Autodesk Fusion 360 part; units mm, degrees
(part 7 of 7)
  spline S25 degree 3 poles (-97.5, 187.4565) (-97.1129, 187.1804) (-96.7258, 186.9044) (-96.3387, 186.6283) (-94.9048, 185.6057) (-93.8881, 184.0523) (-93.1468, 182.2521) (-92.4554, 180.5733) (-91.9675, 178.6373) (-91.4195, 176.7225) (-91.0808, 175.5389) (-90.7149, 174.3638) (-90.3326, 173.4325) (-90.2208, 173.1603) (-90.1088, 172.9111) (-90, 172.6931) knots -1.056001 -1.056001 -1.056001 -1.056001 -1 -1 -1 -0.851292 -0.851292 -0.851292 -0.71262 -0.71262 -0.71262 -0.626906 -0.626906 -0.626906 -0.601856 -0.601856 -0.601856 -0.601856
  spline S26 degree 3 poles (-90, 172.6931) (-89.5881, 173.5183) (-89.1514, 174.7828) (-88.7668, 176.0817) (-88.2129, 177.9522) (-87.737, 179.9069) (-87.1002, 181.6203) (-86.4085, 183.4814) (-85.486, 185.1149) (-84.1355, 186.2591) (-83.9823, 186.3889) (-83.8242, 186.5122) (-83.6613, 186.6283) (-83.2742, 186.9044) (-82.8871, 187.1804) (-82.5, 187.4565) knots -0.398144 -0.398144 -0.398144 -0.398144 -0.30293 -0.30293 -0.30293 -0.165823 -0.165823 -0.165823 -0.016893 -0.016893 -0.016893 0 0 0 0.056001 0.056001 0.056001 0.056001
  spline S27 degree 3 poles (-82.5, 187.4565) (-82.1129, 187.1804) (-81.7258, 186.9044) (-81.3387, 186.6283) (-79.9048, 185.6057) (-78.8881, 184.0523) (-78.1468, 182.2521) (-77.4554, 180.5733) (-76.9675, 178.6373) (-76.4195, 176.7225) (-76.0808, 175.5389) (-75.7149, 174.3638) (-75.3326, 173.4325) (-75.2208, 173.1603) (-75.1088, 172.9111) (-75, 172.6931) knots -1.056001 -1.056001 -1.056001 -1.056001 -1 -1 -1 -0.851292 -0.851292 -0.851292 -0.71262 -0.71262 -0.71262 -0.626906 -0.626906 -0.626906 -0.601856 -0.601856 -0.601856 -0.601856
  spline S28 degree 3 poles (-75, 172.6931) (-74.5881, 173.5183) (-74.1514, 174.7828) (-73.7668, 176.0817) (-73.2129, 177.9522) (-72.737, 179.9069) (-72.1002, 181.6203) (-71.4085, 183.4814) (-70.486, 185.1149) (-69.1355, 186.2591) (-68.9823, 186.3889) (-68.8242, 186.5122) (-68.6613, 186.6283) (-68.2742, 186.9044) (-67.8871, 187.1804) (-67.5, 187.4565) knots -0.398144 -0.398144 -0.398144 -0.398144 -0.30293 -0.30293 -0.30293 -0.165823 -0.165823 -0.165823 -0.016893 -0.016893 -0.016893 0 0 0 0.056001 0.056001 0.056001 0.056001
  spline S29 degree 3 poles (-67.5, 187.4565) (-67.1129, 187.1804) (-66.7258, 186.9044) (-66.3387, 186.6283) (-64.9048, 185.6057) (-63.8881, 184.0523) (-63.1468, 182.2521) (-62.4554, 180.5733) (-61.9675, 178.6373) (-61.4195, 176.7225) (-61.0808, 175.5389) (-60.7149, 174.3638) (-60.3326, 173.4325) (-60.2208, 173.1603) (-60.1088, 172.9111) (-60, 172.6931) knots -1.056001 -1.056001 -1.056001 -1.056001 -1 -1 -1 -0.851292 -0.851292 -0.851292 -0.71262 -0.71262 -0.71262 -0.626906 -0.626906 -0.626906 -0.601856 -0.601856 -0.601856 -0.601856
  spline S30 degree 3 poles (-60, 172.6931) (-59.5881, 173.5183) (-59.1514, 174.7828) (-58.7668, 176.0817) (-58.2129, 177.9522) (-57.737, 179.9069) (-57.1002, 181.6203) (-56.4085, 183.4814) (-55.486, 185.1149) (-54.1355, 186.2591) (-53.9823, 186.3889) (-53.8242, 186.5122) (-53.6613, 186.6283) (-53.2742, 186.9044) (-52.8871, 187.1804) (-52.5, 187.4565) knots -0.398144 -0.398144 -0.398144 -0.398144 -0.30293 -0.30293 -0.30293 -0.165823 -0.165823 -0.165823 -0.016893 -0.016893 -0.016893 0 0 0 0.056001 0.056001 0.056001 0.056001
  spline S31 degree 3 poles (-52.5, 187.4565) (-52.1129, 187.1804) (-51.7258, 186.9044) (-51.3387, 186.6283) (-49.9048, 185.6057) (-48.8881, 184.0523) (-48.1468, 182.2521) (-47.4554, 180.5733) (-46.9675, 178.6373) (-46.4195, 176.7225) (-46.0808, 175.5389) (-45.7149, 174.3638) (-45.3326, 173.4325) (-45.2208, 173.1603) (-45.1088, 172.9111) (-45, 172.6931) knots -1.056001 -1.056001 -1.056001 -1.056001 -1 -1 -1 -0.851292 -0.851292 -0.851292 -0.71262 -0.71262 -0.71262 -0.626906 -0.626906 -0.626906 -0.601856 -0.601856 -0.601856 -0.601856
  spline S32 degree 3 poles (-45, 172.6931) (-44.5881, 173.5183) (-44.1514, 174.7828) (-43.7668, 176.0817) (-43.2129, 177.9522) (-42.737, 179.9069) (-42.1002, 181.6203) (-41.4085, 183.4814) (-40.486, 185.1149) (-39.1355, 186.2591) (-38.9823, 186.3889) (-38.8242, 186.5122) (-38.6613, 186.6283) (-38.2742, 186.9044) (-37.8871, 187.1804) (-37.5, 187.4565) knots -0.398144 -0.398144 -0.398144 -0.398144 -0.30293 -0.30293 -0.30293 -0.165823 -0.165823 -0.165823 -0.016893 -0.016893 -0.016893 0 0 0 0.056001 0.056001 0.056001 0.056001
  spline S33 degree 3 poles (-37.5, 187.4565) (-37.1129, 187.1804) (-36.7258, 186.9044) (-36.3387, 186.6283) (-34.9048, 185.6057) (-33.8881, 184.0523) (-33.1468, 182.2521) (-32.4554, 180.5733) (-31.9675, 178.6373) (-31.4195, 176.7225) (-31.0808, 175.5389) (-30.7149, 174.3638) (-30.3326, 173.4325) (-30.2208, 173.1603) (-30.1088, 172.9111) (-30, 172.6931) knots -1.056001 -1.056001 -1.056001 -1.056001 -1 -1 -1 -0.851292 -0.851292 -0.851292 -0.71262 -0.71262 -0.71262 -0.626906 -0.626906 -0.626906 -0.601856 -0.601856 -0.601856 -0.601856
  spline S34 degree 3 poles (-30, 172.6931) (-29.5881, 173.5183) (-29.1514, 174.7828) (-28.7668, 176.0817) (-28.2129, 177.9522) (-27.737, 179.9069) (-27.1002, 181.6203) (-26.4085, 183.4814) (-25.486, 185.1149) (-24.1355, 186.2591) (-23.9823, 186.3889) (-23.8242, 186.5122) (-23.6613, 186.6283) (-23.2742, 186.9044) (-22.8871, 187.1804) (-22.5, 187.4565) knots -0.398144 -0.398144 -0.398144 -0.398144 -0.30293 -0.30293 -0.30293 -0.165823 -0.165823 -0.165823 -0.016893 -0.016893 -0.016893 0 0 0 0.056001 0.056001 0.056001 0.056001
  spline S35 degree 3 poles (-22.5, 187.4565) (-22.1129, 187.1804) (-21.7258, 186.9044) (-21.3387, 186.6283) (-19.9048, 185.6057) (-18.8881, 184.0523) (-18.1468, 182.2521) (-17.4554, 180.5733) (-16.9675, 178.6373) (-16.4195, 176.7225) (-16.0808, 175.5389) (-15.7149, 174.3638) (-15.3326, 173.4325) (-15.2208, 173.1603) (-15.1088, 172.9111) (-15, 172.6931) knots -1.056001 -1.056001 -1.056001 -1.056001 -1 -1 -1 -0.851292 -0.851292 -0.851292 -0.71262 -0.71262 -0.71262 -0.626906 -0.626906 -0.626906 -0.601856 -0.601856 -0.601856 -0.601856
  spline S36 degree 3 poles (-15, 172.6931) (-14.5881, 173.5183) (-14.1514, 174.7828) (-13.7668, 176.0817) (-13.2129, 177.9522) (-12.737, 179.9069) (-12.1002, 181.6203) (-11.4085, 183.4814) (-10.486, 185.1149) (-9.1355, 186.2591) (-8.9823, 186.3889) (-8.8242, 186.5122) (-8.6613, 186.6283) (-8.3132, 186.8766) (-7.9651, 187.1248) (-7.617, 187.373) knots -0.398144 -0.398144 -0.398144 -0.398144 -0.30293 -0.30293 -0.30293 -0.165823 -0.165823 -0.165823 -0.016893 -0.016893 -0.016893 0 0 0 0.050358 0.050358 0.050358 0.050358
  spline S37 degree 3 poles (-7.617, 187.373) (-7.2462, 187.1603) (-6.8754, 186.9475) (-6.5046, 186.7347) (-5.2151, 185.9947) (-4.3039, 184.7655) (-3.6048, 183.3087) (-2.8011, 181.6339) (-2.2507, 179.5682) (-1.7098, 177.6284) (-1.2417, 175.9499) (-0.7704, 174.4203) (-0.2813, 173.406) (-0.187, 173.2104) (-0.0921, 173.0312) (0, 172.8729) knots -1.111911 -1.111911 -1.111911 -1.111911 -1 -1 -1 -0.758412 -0.758412 -0.758412 -0.480677 -0.480677 -0.480677 -0.240338 -0.240338 -0.240338 -0.19401 -0.19401 -0.19401 -0.19401
  line L6 (-115.3743, 184.93) -> (-124.6275, 184.93)
  spline S38 degree 3 poles (-124.6275, 184.93) (-124.0368, 184.1413) (-123.5509, 183.2334) (-123.1468, 182.2521) (-122.4554, 180.5733) (-121.9675, 178.6373) (-121.4195, 176.7225) (-121.0808, 175.5389) (-120.7149, 174.3638) (-120.3326, 173.4325) (-120.2208, 173.1603) (-120.1088, 172.9111) (-120, 172.6931) knots -0.932352 -0.932352 -0.932352 -0.932352 -0.851292 -0.851292 -0.851292 -0.71262 -0.71262 -0.71262 -0.626906 -0.626906 -0.626906 -0.601856 -0.601856 -0.601856 -0.601856
  arc A1 (-110.6762, 186.0926) -> (-107.3273, 195.8823) centre (-110.5, 191.5) ccw
  spline S39 degree 3 poles (-110.6762, 186.0926) (-109.5836, 185.0976) (-108.7684, 183.7616) (-108.1468, 182.2521) (-107.4554, 180.5733) (-106.9675, 178.6373) (-106.4195, 176.7225) (-106.0808, 175.5389) (-105.7149, 174.3638) (-105.3326, 173.4325) (-105.2208, 173.1603) (-105.1088, 172.9111) (-105, 172.6931) knots -0.975988 -0.975988 -0.975988 -0.975988 -0.851292 -0.851292 -0.851292 -0.71262 -0.71262 -0.71262 -0.626906 -0.626906 -0.626906 -0.601856 -0.601856 -0.601856 -0.601856
  spline S40 degree 3 poles (-120, 172.6931) (-119.5881, 173.5183) (-119.1514, 174.7828) (-118.7668, 176.0817) (-118.2129, 177.9522) (-117.737, 179.9069) (-117.1002, 181.6203) (-116.6441, 182.8475) (-116.0877, 183.9757) (-115.3744, 184.93) knots -0.398144 -0.398144 -0.398144 -0.398144 -0.30293 -0.30293 -0.30293 -0.165823 -0.165823 -0.165823 -0.067621 -0.067621 -0.067621 -0.067621
  spline S41 degree 3 poles (7.617, 187.373) (7.2462, 187.1603) (6.8754, 186.9475) (6.5046, 186.7347) (5.2151, 185.9947) (4.3039, 184.7655) (3.6048, 183.3087) (2.8011, 181.6339) (2.2507, 179.5682) (1.7098, 177.6284) (1.2417, 175.9499) (0.7704, 174.4203) (0.2813, 173.406) (0.187, 173.2104) (0.0921, 173.0312) (0, 172.8729) knots -1.111911 -1.111911 -1.111911 -1.111911 -1 -1 -1 -0.758412 -0.758412 -0.758412 -0.480677 -0.480677 -0.480677 -0.240338 -0.240338 -0.240338 -0.19401 -0.19401 -0.19401 -0.19401
  spline S42 degree 3 poles (15, 172.6931) (14.5881, 173.5183) (14.1514, 174.7828) (13.7668, 176.0817) (13.2129, 177.9522) (12.737, 179.9069) (12.1002, 181.6203) (11.4085, 183.4814) (10.486, 185.1149) (9.1355, 186.2591) (8.9823, 186.3889) (8.8242, 186.5122) (8.6613, 186.6283) (8.3132, 186.8766) (7.9651, 187.1248) (7.617, 187.373) knots -0.398144 -0.398144 -0.398144 -0.398144 -0.30293 -0.30293 -0.30293 -0.165823 -0.165823 -0.165823 -0.016893 -0.016893 -0.016893 0 0 0 0.050358 0.050358 0.050358 0.050358
  spline S43 degree 3 poles (22.5, 187.4565) (22.1129, 187.1804) (21.7258, 186.9044) (21.3387, 186.6283) (19.9048, 185.6057) (18.8881, 184.0523) (18.1468, 182.2521) (17.4554, 180.5733) (16.9675, 178.6373) (16.4195, 176.7225) (16.0808, 175.5389) (15.7149, 174.3638) (15.3326, 173.4325) (15.2208, 173.1603) (15.1088, 172.9111) (15, 172.6931) knots -1.056001 -1.056001 -1.056001 -1.056001 -1 -1 -1 -0.851292 -0.851292 -0.851292 -0.71262 -0.71262 -0.71262 -0.626906 -0.626906 -0.626906 -0.601856 -0.601856 -0.601856 -0.601856
  spline S44 degree 3 poles (30, 172.6931) (29.5881, 173.5183) (29.1514, 174.7828) (28.7668, 176.0817) (28.2129, 177.9522) (27.737, 179.9069) (27.1002, 181.6203) (26.4085, 183.4814) (25.486, 185.1149) (24.1355, 186.2591) (23.9823, 186.3889) (23.8242, 186.5122) (23.6613, 186.6283) (23.2742, 186.9044) (22.8871, 187.1804) (22.5, 187.4565) knots -0.398144 -0.398144 -0.398144 -0.398144 -0.30293 -0.30293 -0.30293 -0.165823 -0.165823 -0.165823 -0.016893 -0.016893 -0.016893 0 0 0 0.056001 0.056001 0.056001 0.056001
  spline S45 degree 3 poles (37.5, 187.4565) (37.1129, 187.1804) (36.7258, 186.9044) (36.3387, 186.6283) (34.9048, 185.6057) (33.8881, 184.0523) (33.1468, 182.2521) (32.4554, 180.5733) (31.9675, 178.6373) (31.4195, 176.7225) (31.0808, 175.5389) (30.7149, 174.3638) (30.3326, 173.4325) (30.2208, 173.1603) (30.1088, 172.9111) (30, 172.6931) knots -1.056001 -1.056001 -1.056001 -1.056001 -1 -1 -1 -0.851292 -0.851292 -0.851292 -0.71262 -0.71262 -0.71262 -0.626906 -0.626906 -0.626906 -0.601856 -0.601856 -0.601856 -0.601856
  spline S46 degree 3 poles (45, 172.6931) (44.5881, 173.5183) (44.1514, 174.7828) (43.7668, 176.0817) (43.2129, 177.9522) (42.737, 179.9069) (42.1002, 181.6203) (41.4085, 183.4814) (40.486, 185.1149) (39.1355, 186.2591) (38.9823, 186.3889) (38.8242, 186.5122) (38.6613, 186.6283) (38.2742, 186.9044) (37.8871, 187.1804) (37.5, 187.4565) knots -0.398144 -0.398144 -0.398144 -0.398144 -0.30293 -0.30293 -0.30293 -0.165823 -0.165823 -0.165823 -0.016893 -0.016893 -0.016893 0 0 0 0.056001 0.056001 0.056001 0.056001
  spline S47 degree 3 poles (52.5, 187.4565) (52.1129, 187.1804) (51.7258, 186.9044) (51.3387, 186.6283) (49.9048, 185.6057) (48.8881, 184.0523) (48.1468, 182.2521) (47.4554, 180.5733) (46.9675, 178.6373) (46.4195, 176.7225) (46.0808, 175.5389) (45.7149, 174.3638) (45.3326, 173.4325) (45.2208, 173.1603) (45.1088, 172.9111) (45, 172.6931) knots -1.056001 -1.056001 -1.056001 -1.056001 -1 -1 -1 -0.851292 -0.851292 -0.851292 -0.71262 -0.71262 -0.71262 -0.626906 -0.626906 -0.626906 -0.601856 -0.601856 -0.601856 -0.601856
  spline S48 degree 3 poles (60, 172.6931) (59.5881, 173.5183) (59.1514, 174.7828) (58.7668, 176.0817) (58.2129, 177.9522) (57.737, 179.9069) (57.1002, 181.6203) (56.4085, 183.4814) (55.486, 185.1149) (54.1355, 186.2591) (53.9823, 186.3889) (53.8242, 186.5122) (53.6613, 186.6283) (53.2742, 186.9044) (52.8871, 187.1804) (52.5, 187.4565) knots -0.398144 -0.398144 -0.398144 -0.398144 -0.30293 -0.30293 -0.30293 -0.165823 -0.165823 -0.165823 -0.016893 -0.016893 -0.016893 0 0 0 0.056001 0.056001 0.056001 0.056001
  spline S49 degree 3 poles (67.5, 187.4565) (67.1129, 187.1804) (66.7258, 186.9044) (66.3387, 186.6283) (64.9048, 185.6057) (63.8881, 184.0523) (63.1468, 182.2521) (62.4554, 180.5733) (61.9675, 178.6373) (61.4195, 176.7225) (61.0808, 175.5389) (60.7149, 174.3638) (60.3326, 173.4325) (60.2208, 173.1603) (60.1088, 172.9111) (60, 172.6931) knots -1.056001 -1.056001 -1.056001 -1.056001 -1 -1 -1 -0.851292 -0.851292 -0.851292 -0.71262 -0.71262 -0.71262 -0.626906 -0.626906 -0.626906 -0.601856 -0.601856 -0.601856 -0.601856
  spline S50 degree 3 poles (75, 172.6931) (74.5881, 173.5183) (74.1514, 174.7828) (73.7668, 176.0817) (73.2129, 177.9522) (72.737, 179.9069) (72.1002, 181.6203) (71.4085, 183.4814) (70.486, 185.1149) (69.1355, 186.2591) (68.9823, 186.3889) (68.8242, 186.5122) (68.6613, 186.6283) (68.2742, 186.9044) (67.8871, 187.1804) (67.5, 187.4565) knots -0.398144 -0.398144 -0.398144 -0.398144 -0.30293 -0.30293 -0.30293 -0.165823 -0.165823 -0.165823 -0.016893 -0.016893 -0.016893 0 0 0 0.056001 0.056001 0.056001 0.056001
  spline S51 degree 3 poles (82.5, 187.4565) (82.1129, 187.1804) (81.7258, 186.9044) (81.3387, 186.6283) (79.9048, 185.6057) (78.8881, 184.0523) (78.1468, 182.2521) (77.4554, 180.5733) (76.9675, 178.6373) (76.4195, 176.7225) (76.0808, 175.5389) (75.7149, 174.3638) (75.3326, 173.4325) (75.2208, 173.1603) (75.1088, 172.9111) (75, 172.6931) knots -1.056001 -1.056001 -1.056001 -1.056001 -1 -1 -1 -0.851292 -0.851292 -0.851292 -0.71262 -0.71262 -0.71262 -0.626906 -0.626906 -0.626906 -0.601856 -0.601856 -0.601856 -0.601856
  spline S52 degree 3 poles (90, 172.6931) (89.5881, 173.5183) (89.1514, 174.7828) (88.7668, 176.0817) (88.2129, 177.9522) (87.737, 179.9069) (87.1002, 181.6203) (86.4085, 183.4814) (85.486, 185.1149) (84.1355, 186.2591) (83.9823, 186.3889) (83.8242, 186.5122) (83.6613, 186.6283) (83.2742, 186.9044) (82.8871, 187.1804) (82.5, 187.4565) knots -0.398144 -0.398144 -0.398144 -0.398144 -0.30293 -0.30293 -0.30293 -0.165823 -0.165823 -0.165823 -0.016893 -0.016893 -0.016893 0 0 0 0.056001 0.056001 0.056001 0.056001
  spline S53 degree 3 poles (97.5, 187.4565) (97.1129, 187.1804) (96.7258, 186.9044) (96.3387, 186.6283) (94.9048, 185.6057) (93.8881, 184.0523) (93.1468, 182.2521) (92.4554, 180.5733) (91.9675, 178.6373) (91.4195, 176.7225) (91.0808, 175.5389) (90.7149, 174.3638) (90.3326, 173.4325) (90.2208, 173.1603) (90.1088, 172.9111) (90, 172.6931) knots -1.056001 -1.056001 -1.056001 -1.056001 -1 -1 -1 -0.851292 -0.851292 -0.851292 -0.71262 -0.71262 -0.71262 -0.626906 -0.626906 -0.626906 -0.601856 -0.601856 -0.601856 -0.601856
  spline S54 degree 3 poles (105, 172.6931) (104.5881, 173.5183) (104.1514, 174.7828) (103.7668, 176.0817) (103.2129, 177.9522) (102.737, 179.9069) (102.1002, 181.6203) (101.4085, 183.4814) (100.486, 185.1149) (99.1355, 186.2591) (98.9823, 186.3889) (98.8242, 186.5122) (98.6613, 186.6283) (98.2742, 186.9044) (97.8871, 187.1804) (97.5, 187.4565) knots -0.398144 -0.398144 -0.398144 -0.398144 -0.30293 -0.30293 -0.30293 -0.165823 -0.165823 -0.165823 -0.016893 -0.016893 -0.016893 0 0 0 0.056001 0.056001 0.056001 0.056001
  spline S55 degree 3 poles (110.6762, 186.0926) (109.5836, 185.0976) (108.7684, 183.7616) (108.1468, 182.2521) (107.4554, 180.5733) (106.9675, 178.6373) (106.4195, 176.7225) (106.0808, 175.5389) (105.7149, 174.3638) (105.3326, 173.4325) (105.2208, 173.1603) (105.1088, 172.9111) (105, 172.6931) knots -0.975988 -0.975988 -0.975988 -0.975988 -0.851292 -0.851292 -0.851292 -0.71262 -0.71262 -0.71262 -0.626906 -0.626906 -0.626906 -0.601856 -0.601856 -0.601856 -0.601856
  arc A2 (107.5392, 196.4416) -> (110.6762, 186.0926) centre (110.3645, 191.6481) ccw
  line L7 (115.3743, 184.93) -> (124.6275, 184.93)
  spline S56 degree 3 poles (120, 172.6931) (119.5881, 173.5183) (119.1514, 174.7828) (118.7668, 176.0817) (118.2129, 177.9522) (117.737, 179.9069) (117.1002, 181.6203) (116.6441, 182.8475) (116.0877, 183.9757) (115.3744, 184.93) knots -0.398144 -0.398144 -0.398144 -0.398144 -0.30293 -0.30293 -0.30293 -0.165823 -0.165823 -0.165823 -0.067621 -0.067621 -0.067621 -0.067621
  spline S57 degree 3 poles (124.6275, 184.93) (124.0368, 184.1413) (123.5509, 183.2334) (123.1468, 182.2521) (122.4554, 180.5733) (121.9675, 178.6373) (121.4195, 176.7225) (121.0808, 175.5389) (120.7149, 174.3638) (120.3326, 173.4325) (120.2208, 173.1603) (120.1088, 172.9111) (120, 172.6931) knots -0.932352 -0.932352 -0.932352 -0.932352 -0.851292 -0.851292 -0.851292 -0.71262 -0.71262 -0.71262 -0.626906 -0.626906 -0.626906 -0.601856 -0.601856 -0.601856 -0.601856
  arc A3 (114.5532, 190.4992) -> (109.4466, 190.4992) centre (111.9999, 190.0086) ccw
  line L8 (114.5532, 190.4992) -> (118.5532, 190.4992)
  arc A4 (118.5532, 189.4992) -> (118.5532, 190.4992) centre (118.5532, 189.9992) ccw
  line L9 (118.5532, 189.4992) -> (114.5532, 189.4992)
  arc A5 (109.4467, 189.4992) -> (114.5532, 189.4992) centre (112, 189.9897) ccw
  line L10 (109.4467, 189.4992) -> (107.4467, 189.4992)
  arc A6 (107.4467, 190.4992) -> (107.4467, 189.4992) centre (107.4467, 189.9992) ccw
  line L11 (107.4467, 190.4992) -> (109.4466, 190.4992)
  arc A7 (-130.5532, 189.508) -> (-125.4467, 189.508) centre (-128, 189.9985) ccw
  line L12 (-130.5532, 189.508) -> (-131.9907, 189.5094)
  arc A8 (-131.9907, 190.4906) -> (-131.9907, 189.5094) centre (-132, 190) ccw
  line L13 (-131.9907, 190.4906) -> (-130.5533, 190.4891)
  arc A9 (-125.4466, 190.4891) -> (-130.5533, 190.4891) centre (-128, 189.9985) ccw
  constraint horizontal L6
  constraint coincident L6 S38.start
  constraint coincident S1 A1.end
  constraint coincident L6 S40.end
  constraint coincident S0 A2.start
sketch "スケッチ15" plane through (0, 0, 15) normal (0, 0, 1) x (-1, 0, 0)
  spline S0 degree 5 poles (122, 185.5) (121.8335, 185.5833) (121.473, 185.7304) (120.8416, 185.9078) (119.7898, 186.0951) (118.3761, 186.0495) (117.1579, 185.4923) (116.4241, 184.2352) (116.286, 182.3186) (116.6933, 179.9858) (117.4973, 177.59) (118.4971, 175.5261) (119.4944, 174.1493) (120.3364, 173.7076) (120.9822, 174.2462) (121.5046, 175.5874) (122.0144, 177.4333) (122.5625, 179.4502) (123.1368, 181.3315) (123.4124, 182.9357) (123.2518, 184.188) (122.8554, 184.8798) (122.4719, 185.231) (122.1665, 185.4168) (122, 185.5) knots 0 0 0 0 0 0 0.05 0.1 0.15 0.2 0.25 0.3 0.35 0.4 0.45 0.5 0.55 0.6 0.65 0.7 0.75 0.8 0.85 0.9 0.95 1 1 1 1 1 1
  line L0 (123, 185) -> (121, 186)
  line L1 (122.5, 179) -> (123.5, 183)
  spline S1 degree 5 poles (-122.0307, 185.5) (-121.8642, 185.5833) (-121.5037, 185.7304) (-120.8723, 185.9078) (-119.8205, 186.0951) (-118.4068, 186.0495) (-117.1886, 185.4923) (-116.4548, 184.2352) (-116.3167, 182.3186) (-116.724, 179.9858) (-117.528, 177.59) (-118.5278, 175.5261) (-119.5251, 174.1493) (-120.3671, 173.7076) (-121.0129, 174.2462) (-121.5354, 175.5874) (-122.0452, 177.4333) (-122.5932, 179.4502) (-123.1675, 181.3315) (-123.4431, 182.9357) (-123.2825, 184.188) (-122.8861, 184.8798) (-122.5027, 185.231) (-122.1972, 185.4168) (-122.0307, 185.5) knots 0 0 0 0 0 0 0.05 0.1 0.15 0.2 0.25 0.3 0.35 0.4 0.45 0.5 0.55 0.6 0.65 0.7 0.75 0.8 0.85 0.9 0.95 1 1 1 1 1 1
  line L2 (-123.0307, 185) -> (-121.0307, 186)
  line L3 (-122.5307, 179) -> (-123.5307, 183)
  arc A0 (107.4467, 190.4992) -> (107.4467, 189.4992) centre (107.4467, 189.9992) ccw
  arc A1 (114.5532, 190.4992) -> (109.4466, 190.4992) centre (111.9999, 190.0086) ccw
  line L4 (114.5532, 190.4992) -> (118.5532, 190.4992)
  arc A2 (118.5532, 189.4992) -> (118.5532, 190.4992) centre (118.5532, 189.9992) ccw
  line L5 (118.5532, 189.4992) -> (114.5532, 189.4992)
  arc A3 (109.4467, 189.4992) -> (114.5532, 189.4992) centre (112, 189.9897) ccw
  line L6 (109.4467, 189.4992) -> (107.4467, 189.4992)
  line L7 (107.4467, 190.4992) -> (109.4466, 190.4992)
  arc A4 (-130.5532, 189.508) -> (-125.4467, 189.508) centre (-128, 189.9985) ccw
  line L8 (-130.5532, 189.508) -> (-131.9907, 189.5094)
  arc A5 (-131.9907, 190.4906) -> (-131.9907, 189.5094) centre (-132, 190) ccw
  line L9 (-131.9907, 190.4906) -> (-130.5533, 190.4891)
  arc A6 (-125.4466, 190.4891) -> (-130.5533, 190.4891) centre (-128, 189.9985) ccw
  line L10 (-125.4466, 190.4891) -> (-118.5, 190.4891)
  arc A7 (-118.5, 189.508) -> (-118.5, 190.4891) centre (-118.4907, 189.9985) ccw
  line L11 (-118.5, 189.508) -> (-125.4467, 189.508)
  line L12 (111.2071, 197) -> (110, 197)
  spline S2 degree 5 poles (110, 197) (109.531, 197) (108.6035, 196.8979) (107.2432, 196.4388) (105.4719, 195.335) (103.2255, 193.665) (101.2961, 192.5612) (99.7118, 192.1021) (98.5828, 192) (98, 192) knots 0 0 0 0 0 0 0.2 0.4 0.6 0.8 1 1 1 1 1 1
  line L13 (98, 192) -> (-98, 192)
  spline S3 degree 5 poles (-98, 192) (-98.3058, 192) (-98.9114, 192.0121) (-99.802, 192.0667) (-100.9513, 192.2172) (-102.3121, 192.5594) (-103.5836, 193.0784) (-104.7577, 193.7777) (-105.839, 194.6251) (-106.8563, 195.5224) (-107.855, 196.3282) (-108.6773, 196.7819) (-109.3246, 196.9603) (-109.7722, 197) (-110, 197) knots -1 -1 -1 -1 -1 -1 -0.9 -0.8 -0.7 -0.6 -0.5 -0.4 -0.3 -0.2 -0.1 0 0 0 0 0 0
  line L14 (-110, 197) -> (-124.5, 197)
  spline S4 degree 5 poles (-124.5, 197) (-124.9971, 197) (-125.9797, 196.9323) (-127.4185, 196.6274) (-129.2284, 195.8334) (-131.112, 194.3075) (-132.4303, 192.406) (-133.077, 190.3015) (-133.1999, 188.1805) (-133.1301, 186.1742) (-133.012, 184.2924) (-132.951, 182.4907) (-132.9863, 180.6906) (-133.1364, 178.8191) (-133.409, 176.8339) (-133.8064, 174.7125) (-134.2233, 172.8999) (-134.5905, 171.4751) (-134.8595, 170.4965) (-135, 170) knots 0 0 0 0 0 0 0.066667 0.133333 0.2 0.266667 0.333333 0.4 0.466667 0.533333 0.6 0.666667 0.733333 0.8 0.866667 0.933333 1 1 1 1 1 1
  spline S5 degree 5 poles (-135, 170) (-134.8788, 170) (-134.6377, 170.0414) (-134.2795, 170.2276) (-133.8109, 170.7132) (-133.2504, 171.6514) (-132.7264, 172.8364) (-132.2468, 174.1779) (-131.811, 175.5961) (-131.4086, 177.0279) (-131.0241, 178.4225) (-130.6386, 179.7408) (-130.2334, 180.9541) (-129.7917, 182.0427) (-129.3023, 182.9962) (-128.7602, 183.8116) (-128.2831, 184.3542) (-127.9009, 184.7005) (-127.6354, 184.9046) (-127.5, 185) knots -1 -1 -1 -1 -1 -1 -0.933333 -0.866667 -0.8 -0.733333 -0.666667 -0.6 -0.533333 -0.466667 -0.4 -0.333333 -0.266667 -0.2 -0.133333 -0.066667 0 0 0 0 0 0
  spline S6 degree 5 poles (-127.5, 185) (-127.3618, 184.9014) (-127.0912, 184.691) (-126.7034, 184.3357) (-126.2221, 183.7824) (-125.6794, 182.9585) (-125.1925, 182.0039) (-124.7547, 180.9239) (-124.3537, 179.7274) (-123.9726, 178.4298) (-123.5928, 177.0547) (-123.1957, 175.6366) (-122.7655, 174.223) (-122.2912, 172.8764) (-121.7698, 171.6789) (-121.2063, 170.7262) (-120.6114, 170.1082) (-120, 169.8927) (-119.3886, 170.1082) (-118.7937, 170.7262) (-118.2302, 171.6789) (-117.7088, 172.8764) (-117.2345, 174.223) (-116.8043, 175.6366) (-116.4072, 177.0547) (-116.0274, 178.4298) (-115.6463, 179.7274) (-115.2453, 180.9239) (-114.8075, 182.0039) (-114.3206, 182.9585) (-113.7779, 183.7824) (-113.2966, 184.3357) (-112.9088, 184.691) (-112.6382, 184.9014) (-112.5, 185) knots -1 -1 -1 -1 -1 -1 -0.966667 -0.933333 -0.9 -0.866667 -0.833333 -0.8 -0.766667 -0.733333 -0.7 -0.666667 -0.633333 -0.6 -0.566667 -0.533333 -0.5 -0.466667 -0.433333 -0.4 -0.366667 -0.333333 -0.3 -0.266667 -0.233333 -0.2 -0.166667 -0.133333 -0.1 -0.066667 -0.033333 0 0 0 0 0 0
  spline S7 degree 5 poles (-112.5, 185) (-112.3618, 184.9014) (-112.0912, 184.691) (-111.7034, 184.3357) (-111.2221, 183.7824) (-110.6794, 182.9585) (-110.1925, 182.0039) (-109.7547, 180.9239) (-109.3537, 179.7274) (-108.9726, 178.4298) (-108.5928, 177.0547) (-108.1957, 175.6366) (-107.7655, 174.223) (-107.2912, 172.8764) (-106.7698, 171.6789) (-106.2063, 170.7262) (-105.6114, 170.1082) (-105, 169.8927) (-104.3886, 170.1082) (-103.7937, 170.7262) (-103.2302, 171.6789) (-102.7088, 172.8764) (-102.2345, 174.223) (-101.8043, 175.6366) (-101.4072, 177.0547) (-101.0274, 178.4298) (-100.6463, 179.7274) (-100.2453, 180.9239) (-99.8075, 182.0039) (-99.3206, 182.9585) (-98.7779, 183.7824) (-98.2966, 184.3357) (-97.9088, 184.691) (-97.6382, 184.9014) (-97.5, 185) knots -1 -1 -1 -1 -1 -1 -0.966667 -0.933333 -0.9 -0.866667 -0.833333 -0.8 -0.766667 -0.733333 -0.7 -0.666667 -0.633333 -0.6 -0.566667 -0.533333 -0.5 -0.466667 -0.433333 -0.4 -0.366667 -0.333333 -0.3 -0.266667 -0.233333 -0.2 -0.166667 -0.133333 -0.1 -0.066667 -0.033333 0 0 0 0 0 0
  spline S8 degree 5 poles (-97.5, 185) (-97.3618, 184.9014) (-97.0912, 184.691) (-96.7034, 184.3357) (-96.2221, 183.7824) (-95.6794, 182.9585) (-95.1925, 182.0039) (-94.7547, 180.9239) (-94.3537, 179.7274) (-93.9726, 178.4298) (-93.5928, 177.0547) (-93.1957, 175.6366) (-92.7655, 174.223) (-92.2912, 172.8764) (-91.7698, 171.6789) (-91.2063, 170.7262) (-90.6114, 170.1082) (-90, 169.8927) (-89.3886, 170.1082) (-88.7937, 170.7262) (-88.2302, 171.6789) (-87.7088, 172.8764) (-87.2345, 174.223) (-86.8043, 175.6366) (-86.4072, 177.0547) (-86.0274, 178.4298) (-85.6463, 179.7274) (-85.2453, 180.9239) (-84.8075, 182.0039) (-84.3206, 182.9585) (-83.7779, 183.7824) (-83.2966, 184.3357) (-82.9088, 184.691) (-82.6382, 184.9014) (-82.5, 185) knots -1 -1 -1 -1 -1 -1 -0.966667 -0.933333 -0.9 -0.866667 -0.833333 -0.8 -0.766667 -0.733333 -0.7 -0.666667 -0.633333 -0.6 -0.566667 -0.533333 -0.5 -0.466667 -0.433333 -0.4 -0.366667 -0.333333 -0.3 -0.266667 -0.233333 -0.2 -0.166667 -0.133333 -0.1 -0.066667 -0.033333 0 0 0 0 0 0
  spline S9 degree 5 poles (-82.5, 185) (-82.3618, 184.9014) (-82.0912, 184.691) (-81.7034, 184.3357) (-81.2221, 183.7824) (-80.6794, 182.9585) (-80.1925, 182.0039) (-79.7547, 180.9239) (-79.3537, 179.7274) (-78.9726, 178.4298) (-78.5928, 177.0547) (-78.1957, 175.6366) (-77.7655, 174.223) (-77.2912, 172.8764) (-76.7698, 171.6789) (-76.2063, 170.7262) (-75.6114, 170.1082) (-75, 169.8927) (-74.3886, 170.1082) (-73.7937, 170.7262) (-73.2302, 171.6789) (-72.7088, 172.8764) (-72.2345, 174.223) (-71.8043, 175.6366) (-71.4072, 177.0547) (-71.0274, 178.4298) (-70.6463, 179.7274) (-70.2453, 180.9239) (-69.8075, 182.0039) (-69.3206, 182.9585) (-68.7779, 183.7824) (-68.2966, 184.3357) (-67.9088, 184.691) (-67.6382, 184.9014) (-67.5, 185) knots -1 -1 -1 -1 -1 -1 -0.966667 -0.933333 -0.9 -0.866667 -0.833333 -0.8 -0.766667 -0.733333 -0.7 -0.666667 -0.633333 -0.6 -0.566667 -0.533333 -0.5 -0.466667 -0.433333 -0.4 -0.366667 -0.333333 -0.3 -0.266667 -0.233333 -0.2 -0.166667 -0.133333 -0.1 -0.066667 -0.033333 0 0 0 0 0 0
  spline S10 degree 5 poles (-67.5, 185) (-67.3618, 184.9014) (-67.0912, 184.691) (-66.7034, 184.3357) (-66.2221, 183.7824) (-65.6794, 182.9585) (-65.1925, 182.0039) (-64.7547, 180.9239) (-64.3537, 179.7274) (-63.9726, 178.4298) (-63.5928, 177.0547) (-63.1957, 175.6366) (-62.7655, 174.223) (-62.2912, 172.8764) (-61.7698, 171.6789) (-61.2063, 170.7262) (-60.6114, 170.1082) (-60, 169.8927) (-59.3886, 170.1082) (-58.7937, 170.7262) (-58.2302, 171.6789) (-57.7088, 172.8764) (-57.2345, 174.223) (-56.8043, 175.6366) (-56.4072, 177.0547) (-56.0274, 178.4298) (-55.6463, 179.7274) (-55.2453, 180.9239) (-54.8075, 182.0039) (-54.3206, 182.9585) (-53.7779, 183.7824) (-53.2966, 184.3357) (-52.9088, 184.691) (-52.6382, 184.9014) (-52.5, 185) knots -1 -1 -1 -1 -1 -1 -0.966667 -0.933333 -0.9 -0.866667 -0.833333 -0.8 -0.766667 -0.733333 -0.7 -0.666667 -0.633333 -0.6 -0.566667 -0.533333 -0.5 -0.466667 -0.433333 -0.4 -0.366667 -0.333333 -0.3 -0.266667 -0.233333 -0.2 -0.166667 -0.133333 -0.1 -0.066667 -0.033333 0 0 0 0 0 0
  spline S11 degree 5 poles (-52.5, 185) (-52.3618, 184.9014) (-52.0912, 184.691) (-51.7034, 184.3357) (-51.2221, 183.7824) (-50.6794, 182.9585) (-50.1925, 182.0039) (-49.7547, 180.9239) (-49.3537, 179.7274) (-48.9726, 178.4298) (-48.5928, 177.0547) (-48.1957, 175.6366) (-47.7655, 174.223) (-47.2912, 172.8764) (-46.7698, 171.6789) (-46.2063, 170.7262) (-45.6114, 170.1082) (-45, 169.8927) (-44.3886, 170.1082) (-43.7937, 170.7262) (-43.2302, 171.6789) (-42.7088, 172.8764) (-42.2345, 174.223) (-41.8043, 175.6366) (-41.4072, 177.0547) (-41.0274, 178.4298) (-40.6463, 179.7274) (-40.2453, 180.9239) (-39.8075, 182.0039) (-39.3206, 182.9585) (-38.7779, 183.7824) (-38.2966, 184.3357) (-37.9088, 184.691) (-37.6382, 184.9014) (-37.5, 185) knots -1 -1 -1 -1 -1 -1 -0.966667 -0.933333 -0.9 -0.866667 -0.833333 -0.8 -0.766667 -0.733333 -0.7 -0.666667 -0.633333 -0.6 -0.566667 -0.533333 -0.5 -0.466667 -0.433333 -0.4 -0.366667 -0.333333 -0.3 -0.266667 -0.233333 -0.2 -0.166667 -0.133333 -0.1 -0.066667 -0.033333 0 0 0 0 0 0
  spline S12 degree 5 poles (-37.5, 185) (-37.3618, 184.9014) (-37.0912, 184.691) (-36.7034, 184.3357) (-36.2221, 183.7824) (-35.6794, 182.9585) (-35.1925, 182.0039) (-34.7547, 180.9239) (-34.3537, 179.7274) (-33.9726, 178.4298) (-33.5928, 177.0547) (-33.1957, 175.6366) (-32.7655, 174.223) (-32.2912, 172.8764) (-31.7698, 171.6789) (-31.2063, 170.7262) (-30.6114, 170.1082) (-30, 169.8927) (-29.3886, 170.1082) (-28.7937, 170.7262) (-28.2302, 171.6789) (-27.7088, 172.8764) (-27.2345, 174.223) (-26.8043, 175.6366) (-26.4072, 177.0547) (-26.0274, 178.4298) (-25.6463, 179.7274) (-25.2453, 180.9239) (-24.8075, 182.0039) (-24.3206, 182.9585) (-23.7779, 183.7824) (-23.2966, 184.3357) (-22.9088, 184.691) (-22.6382, 184.9014) (-22.5, 185) knots -1 -1 -1 -1 -1 -1 -0.966667 -0.933333 -0.9 -0.866667 -0.833333 -0.8 -0.766667 -0.733333 -0.7 -0.666667 -0.633333 -0.6 -0.566667 -0.533333 -0.5 -0.466667 -0.433333 -0.4 -0.366667 -0.333333 -0.3 -0.266667 -0.233333 -0.2 -0.166667 -0.133333 -0.1 -0.066667 -0.033333 0 0 0 0 0 0
  spline S13 degree 5 poles (-22.5, 185) (-22.3618, 184.9014) (-22.0912, 184.691) (-21.7034, 184.3357) (-21.2221, 183.7824) (-20.6794, 182.9585) (-20.1925, 182.0039) (-19.7547, 180.9239) (-19.3537, 179.7274) (-18.9726, 178.4298) (-18.5928, 177.0547) (-18.1957, 175.6366) (-17.7655, 174.223) (-17.2912, 172.8764) (-16.7698, 171.6789) (-16.2063, 170.7262) (-15.6114, 170.1082) (-15, 169.8927) (-14.3886, 170.1082) (-13.7937, 170.7262) (-13.2302, 171.6789) (-12.7088, 172.8764) (-12.2345, 174.223) (-11.8043, 175.6366) (-11.4072, 177.0547) (-11.0274, 178.4298) (-10.6463, 179.7274) (-10.2453, 180.9239) (-9.8075, 182.0039) (-9.3206, 182.9585) (-8.7779, 183.7824) (-8.2966, 184.3357) (-7.9088, 184.691) (-7.6382, 184.9014) (-7.5, 185) knots -1 -1 -1 -1 -1 -1 -0.966667 -0.933333 -0.9 -0.866667 -0.833333 -0.8 -0.766667 -0.733333 -0.7 -0.666667 -0.633333 -0.6 -0.566667 -0.533333 -0.5 -0.466667 -0.433333 -0.4 -0.366667 -0.333333 -0.3 -0.266667 -0.233333 -0.2 -0.166667 -0.133333 -0.1 -0.066667 -0.033333 0 0 0 0 0 0
  spline S14 degree 5 poles (-7.5, 185) (-7.3675, 184.9239) (-7.1071, 184.754) (-6.7306, 184.4454) (-6.2569, 183.926) (-5.7125, 183.0952) (-5.2148, 182.0863) (-4.7604, 180.9127) (-4.3411, 179.6053) (-3.9444, 178.2117) (-3.5556, 176.7883) (-3.1589, 175.3947) (-2.7396, 174.0873) (-2.2852, 172.9137) (-1.7875, 171.9048) (-1.2431, 171.074) (-0.7694, 170.5546) (-0.3929, 170.246) (-0.1325, 170.0761) (0, 170) knots -1 -1 -1 -1 -1 -1 -0.933333 -0.866667 -0.8 -0.733333 -0.666667 -0.6 -0.533333 -0.466667 -0.4 -0.333333 -0.266667 -0.2 -0.133333 -0.066667 0 0 0 0 0 0
  spline S15 degree 5 poles (0, 170) (0.1325, 170.0761) (0.3929, 170.246) (0.7694, 170.5546) (1.2431, 171.074) (1.7875, 171.9048) (2.2852, 172.9137) (2.7396, 174.0873) (3.1589, 175.3947) (3.5556, 176.7883) (3.9444, 178.2117) (4.3411, 179.6053) (4.7604, 180.9127) (5.2148, 182.0863) (5.7125, 183.0952) (6.2569, 183.926) (6.7306, 184.4454) (7.1071, 184.754) (7.3675, 184.9239) (7.5, 185) knots 0 0 0 0 0 0 0.066667 0.133333 0.2 0.266667 0.333333 0.4 0.466667 0.533333 0.6 0.666667 0.733333 0.8 0.866667 0.933333 1 1 1 1 1 1
  spline S16 degree 5 poles (7.5, 185) (7.6382, 184.9014) (7.9088, 184.691) (8.2966, 184.3357) (8.7779, 183.7824) (9.3206, 182.9585) (9.8075, 182.0039) (10.2453, 180.9239) (10.6463, 179.7274) (11.0274, 178.4298) (11.4072, 177.0547) (11.8043, 175.6366) (12.2345, 174.223) (12.7088, 172.8764) (13.2302, 171.6789) (13.7937, 170.7262) (14.3886, 170.1082) (15, 169.8927) (15.6114, 170.1082) (16.2063, 170.7262) (16.7698, 171.6789) (17.2912, 172.8764) (17.7655, 174.223) (18.1957, 175.6366) (18.5928, 177.0547) (18.9726, 178.4298) (19.3537, 179.7274) (19.7547, 180.9239) (20.1925, 182.0039) (20.6794, 182.9585) (21.2221, 183.7824) (21.7034, 184.3357) (22.0912, 184.691) (22.3618, 184.9014) (22.5, 185) knots 0 0 0 0 0 0 0.033333 0.066667 0.1 0.133333 0.166667 0.2 0.233333 0.266667 0.3 0.333333 0.366667 0.4 0.433333 0.466667 0.5 0.533333 0.566667 0.6 0.633333 0.666667 0.7 0.733333 0.766667 0.8 0.833333 0.866667 0.9 0.933333 0.966667 1 1 1 1 1 1
  spline S17 degree 5 poles (22.5, 185) (22.6382, 184.9014) (22.9088, 184.691) (23.2966, 184.3357) (23.7779, 183.7824) (24.3206, 182.9585) (24.8075, 182.0039) (25.2453, 180.9239) (25.6463, 179.7274) (26.0274, 178.4298) (26.4072, 177.0547) (26.8043, 175.6366) (27.2345, 174.223) (27.7088, 172.8764) (28.2302, 171.6789) (28.7937, 170.7262) (29.3886, 170.1082) (30, 169.8927) (30.6114, 170.1082) (31.2063, 170.7262) (31.7698, 171.6789) (32.2912, 172.8764) (32.7655, 174.223) (33.1957, 175.6366) (33.5928, 177.0547) (33.9726, 178.4298) (34.3537, 179.7274) (34.7547, 180.9239) (35.1925, 182.0039) (35.6794, 182.9585) (36.2221, 183.7824) (36.7034, 184.3357) (37.0912, 184.691) (37.3618, 184.9014) (37.5, 185) knots 0 0 0 0 0 0 0.033333 0.066667 0.1 0.133333 0.166667 0.2 0.233333 0.266667 0.3 0.333333 0.366667 0.4 0.433333 0.466667 0.5 0.533333 0.566667 0.6 0.633333 0.666667 0.7 0.733333 0.766667 0.8 0.833333 0.866667 0.9 0.933333 0.966667 1 1 1 1 1 1
  spline S18 degree 5 poles (37.5, 185) (37.6382, 184.9014) (37.9088, 184.691) (38.2966, 184.3357) (38.7779, 183.7824) (39.3206, 182.9585) (39.8075, 182.0039) (40.2453, 180.9239) (40.6463, 179.7274) (41.0274, 178.4298) (41.4072, 177.0547) (41.8043, 175.6366) (42.2345, 174.223) (42.7088, 172.8764) (43.2302, 171.6789) (43.7937, 170.7262) (44.3886, 170.1082) (45, 169.8927) (45.6114, 170.1082) (46.2063, 170.7262) (46.7698, 171.6789) (47.2912, 172.8764) (47.7655, 174.223) (48.1957, 175.6366) (48.5928, 177.0547) (48.9726, 178.4298) (49.3537, 179.7274) (49.7547, 180.9239) (50.1925, 182.0039) (50.6794, 182.9585) (51.2221, 183.7824) (51.7034, 184.3357) (52.0912, 184.691) (52.3618, 184.9014) (52.5, 185) knots 0 0 0 0 0 0 0.033333 0.066667 0.1 0.133333 0.166667 0.2 0.233333 0.266667 0.3 0.333333 0.366667 0.4 0.433333 0.466667 0.5 0.533333 0.566667 0.6 0.633333 0.666667 0.7 0.733333 0.766667 0.8 0.833333 0.866667 0.9 0.933333 0.966667 1 1 1 1 1 1
  spline S19 degree 5 poles (52.5, 185) (52.6382, 184.9014) (52.9088, 184.691) (53.2966, 184.3357) (53.7779, 183.7824) (54.3206, 182.9585) (54.8075, 182.0039) (55.2453, 180.9239) (55.6463, 179.7274) (56.0274, 178.4298) (56.4072, 177.0547) (56.8043, 175.6366) (57.2345, 174.223) (57.7088, 172.8764) (58.2302, 171.6789) (58.7937, 170.7262) (59.3886, 170.1082) (60, 169.8927) (60.6114, 170.1082) (61.2063, 170.7262) (61.7698, 171.6789) (62.2912, 172.8764) (62.7655, 174.223) (63.1957, 175.6366) (63.5928, 177.0547) (63.9726, 178.4298) (64.3537, 179.7274) (64.7547, 180.9239) (65.1925, 182.0039) (65.6794, 182.9585) (66.2221, 183.7824) (66.7034, 184.3357) (67.0912, 184.691) (67.3618, 184.9014) (67.5, 185) knots 0 0 0 0 0 0 0.033333 0.066667 0.1 0.133333 0.166667 0.2 0.233333 0.266667 0.3 0.333333 0.366667 0.4 0.433333 0.466667 0.5 0.533333 0.566667 0.6 0.633333 0.666667 0.7 0.733333 0.766667 0.8 0.833333 0.866667 0.9 0.933333 0.966667 1 1 1 1 1 1
  spline S20 degree 5 poles (67.5, 185) (67.6382, 184.9014) (67.9088, 184.691) (68.2966, 184.3357) (68.7779, 183.7824) (69.3206, 182.9585) (69.8075, 182.0039) (70.2453, 180.9239) (70.6463, 179.7274) (71.0274, 178.4298) (71.4072, 177.0547) (71.8043, 175.6366) (72.2345, 174.223) (72.7088, 172.8764) (73.2302, 171.6789) (73.7937, 170.7262) (74.3886, 170.1082) (75, 169.8927) (75.6114, 170.1082) (76.2063, 170.7262) (76.7698, 171.6789) (77.2912, 172.8764) (77.7655, 174.223) (78.1957, 175.6366) (78.5928, 177.0547) (78.9726, 178.4298) (79.3537, 179.7274) (79.7547, 180.9239) (80.1925, 182.0039) (80.6794, 182.9585) (81.2221, 183.7824) (81.7034, 184.3357) (82.0912, 184.691) (82.3618, 184.9014) (82.5, 185) knots 0 0 0 0 0 0 0.033333 0.066667 0.1 0.133333 0.166667 0.2 0.233333 0.266667 0.3 0.333333 0.366667 0.4 0.433333 0.466667 0.5 0.533333 0.566667 0.6 0.633333 0.666667 0.7 0.733333 0.766667 0.8 0.833333 0.866667 0.9 0.933333 0.966667 1 1 1 1 1 1
  spline S21 degree 5 poles (82.5, 185) (82.6382, 184.9014) (82.9088, 184.691) (83.2966, 184.3357) (83.7779, 183.7824) (84.3206, 182.9585) (84.8075, 182.0039) (85.2453, 180.9239) (85.6463, 179.7274) (86.0274, 178.4298) (86.4072, 177.0547) (86.8043, 175.6366) (87.2345, 174.223) (87.7088, 172.8764) (88.2302, 171.6789) (88.7937, 170.7262) (89.3886, 170.1082) (90, 169.8927) (90.6114, 170.1082) (91.2063, 170.7262) (91.7698, 171.6789) (92.2912, 172.8764) (92.7655, 174.223) (93.1957, 175.6366) (93.5928, 177.0547) (93.9726, 178.4298) (94.3537, 179.7274) (94.7547, 180.9239) (95.1925, 182.0039) (95.6794, 182.9585) (96.2221, 183.7824) (96.7034, 184.3357) (97.0912, 184.691) (97.3618, 184.9014) (97.5, 185) knots 0 0 0 0 0 0 0.033333 0.066667 0.1 0.133333 0.166667 0.2 0.233333 0.266667 0.3 0.333333 0.366667 0.4 0.433333 0.466667 0.5 0.533333 0.566667 0.6 0.633333 0.666667 0.7 0.733333 0.766667 0.8 0.833333 0.866667 0.9 0.933333 0.966667 1 1 1 1 1 1
  spline S22 degree 5 poles (97.5, 185) (97.6382, 184.9014) (97.9088, 184.691) (98.2966, 184.3357) (98.7779, 183.7824) (99.3206, 182.9585) (99.8075, 182.0039) (100.2453, 180.9239) (100.6463, 179.7274) (101.0274, 178.4298) (101.4072, 177.0547) (101.8043, 175.6366) (102.2345, 174.223) (102.7088, 172.8764) (103.2302, 171.6789) (103.7937, 170.7262) (104.3886, 170.1082) (105, 169.8927) (105.6114, 170.1082) (106.2063, 170.7262) (106.7698, 171.6789) (107.2912, 172.8764) (107.7655, 174.223) (108.1957, 175.6366) (108.5928, 177.0547) (108.9726, 178.4298) (109.3537, 179.7274) (109.7547, 180.9239) (110.1925, 182.0039) (110.6794, 182.9585) (111.2221, 183.7824) (111.7034, 184.3357) (112.0912, 184.691) (112.3618, 184.9014) (112.5, 185) knots 0 0 0 0 0 0 0.033333 0.066667 0.1 0.133333 0.166667 0.2 0.233333 0.266667 0.3 0.333333 0.366667 0.4 0.433333 0.466667 0.5 0.533333 0.566667 0.6 0.633333 0.666667 0.7 0.733333 0.766667 0.8 0.833333 0.866667 0.9 0.933333 0.966667 1 1 1 1 1 1
  spline S23 degree 5 poles (112.5, 185) (112.6382, 184.9014) (112.9088, 184.691) (113.2966, 184.3357) (113.7779, 183.7824) (114.3206, 182.9585) (114.8075, 182.0039) (115.2453, 180.9239) (115.6463, 179.7274) (116.0274, 178.4298) (116.4072, 177.0547) (116.8043, 175.6366) (117.2345, 174.223) (117.7088, 172.8764) (118.2302, 171.6789) (118.7937, 170.7262) (119.3886, 170.1082) (120, 169.8927) (120.6114, 170.1082) (121.2063, 170.7262) (121.7698, 171.6789) (122.2912, 172.8764) (122.7655, 174.223) (123.1957, 175.6366) (123.5928, 177.0547) (123.9726, 178.4298) (124.3537, 179.7274) (124.7547, 180.9239) (125.1925, 182.0039) (125.6794, 182.9585) (126.2221, 183.7824) (126.7034, 184.3357) (127.0912, 184.691) (127.3618, 184.9014) (127.5, 185) knots 0 0 0 0 0 0 0.033333 0.066667 0.1 0.133333 0.166667 0.2 0.233333 0.266667 0.3 0.333333 0.366667 0.4 0.433333 0.466667 0.5 0.533333 0.566667 0.6 0.633333 0.666667 0.7 0.733333 0.766667 0.8 0.833333 0.866667 0.9 0.933333 0.966667 1 1 1 1 1 1
  spline S24 degree 5 poles (127.5, 185) (127.6354, 184.9046) (127.9009, 184.7005) (128.2831, 184.3542) (128.7602, 183.8116) (129.3023, 182.9962) (129.7917, 182.0427) (130.2334, 180.9541) (130.6386, 179.7408) (131.0241, 178.4225) (131.4086, 177.0279) (131.811, 175.5961) (132.2468, 174.1779) (132.7264, 172.8364) (133.2504, 171.6514) (133.8109, 170.7132) (134.2795, 170.2276) (134.6377, 170.0414) (134.8788, 170) (135, 170) knots 0 0 0 0 0 0 0.066667 0.133333 0.2 0.266667 0.333333 0.4 0.466667 0.533333 0.6 0.666667 0.733333 0.8 0.866667 0.933333 1 1 1 1 1 1
  spline S25 degree 5 poles (135, 170) (134.8595, 170.4965) (134.5905, 171.4751) (134.2233, 172.8999) (133.8064, 174.7125) (133.409, 176.8339) (133.1364, 178.8191) (132.9863, 180.6906) (132.951, 182.4907) (133.012, 184.2924) (133.1301, 186.1742) (133.1999, 188.1805) (133.077, 190.3015) (132.4303, 192.406) (131.112, 194.3075) (129.2284, 195.8334) (127.4185, 196.6274) (125.9797, 196.9323) (124.9971, 197) (124.5, 197) knots -1 -1 -1 -1 -1 -1 -0.933333 -0.866667 -0.8 -0.733333 -0.666667 -0.6 -0.533333 -0.466667 -0.4 -0.333333 -0.266667 -0.2 -0.133333 -0.066667 0 0 0 0 0 0
  line L15 (124.5, 197) -> (111.2071, 197)
  point P0 (117, 185)
  point P1 (120, 174)
  point P2 (123, 181)
  point P3 (-123.0307, 181)
  point P4 (-117.0307, 185)
  point P5 (-120.0307, 174)
  constraint midpoint S0.start L0
  constraint midpoint P2 L1
  constraint midpoint S1.start L2
  constraint midpoint P3 L3
extrude "押し出し14" cut sketch "スケッチ15" against normal blind 35 contours S0 | S1
extrude "押し出し16" cut sketch "スケッチ14" against normal blind 10 contours S0 L3 S1 S24 S25 S26 S27 S28 S29 S30 S31 S32 S33 S34 S35 S36 S37 A1 S39 S41 S42 S43 S44 S45 S46 S47 S48 S49 S50 S51 S52 S53 S54 S55 A2
